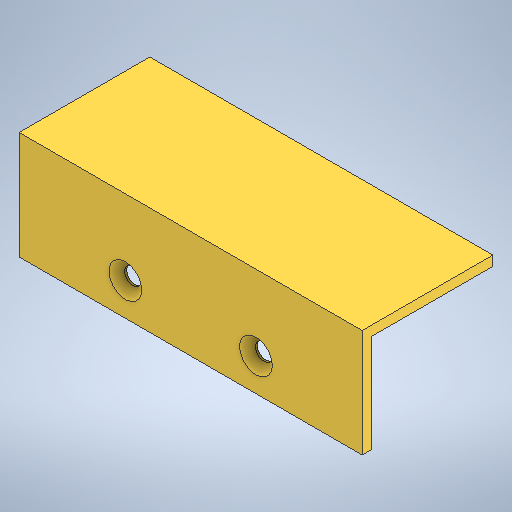
# Autodesk Inventor part: TS_Magazin_Begrenzung_int
Saved by Autodesk Inventor 2025.2 (Build 292293000, 293)
## iProperties
Created: 2025-06-01
Part Number: TS_Magazin_Begrenzung_int
Material: Generisch
Document SubType Name: Modeling
Designer: tino
Density: 1 g/cm^3
Appearance: Vorgabe
Author: tino
Autodesk Inventor part; units mm, degrees
ref_plane "YZ Plane" through (0, 0, 0) normal (1, 0, 0) x (0, 1, 0)
ref_plane "XZ Plane" through (0, 0, 0) normal (0, 1, 0) x (-1, 0, 0)
ref_plane "XY Plane" through (0, 0, 0) normal (0, 0, 1) x (1, 0, 0)
sketch "Skizze1" plane through (0, 0, 0) normal (1, 0, 0) x (0, 1, 0)
  line L0 (0, 0) -> (3, 0)
  line L1 (3, 0) -> (3, 30)
  line L2 (3, 30) -> (0, 30)
  line L3 (0, 30) -> (0, 0)
  line L4 (0, 30) -> (40, 30)
  line L5 (40, 30) -> (40, 33)
  line L6 (40, 33) -> (0, 33)
  line L7 (0, 33) -> (0, 30)
  dimension "d1" = 3
  dimension "d2" = 30
  dimension "d3" = 40
  dimension "d4" = 3
  constraints: 16 end point, 4 parallel, 2 horizontal, 2 perpendicular
  measures "d1" distance of L2.end L1.end
  measures "d2" distance of L1.end L0.end
  measures "d3" distance of L6.end L5.end
  measures "d4" distance between parallel lines of L4 L6
extrude "Extrusion1" add sketch "Skizze1" along normal mid plane 105
sketch "Skizze2" plane through (-52.5, 0, 0) normal (0, -1, 0) x (1, 0, 0)
  line L0 (10.5897, 10) -> (79.1743, 10) construction
  line L1 (0, 0) -> (105, 0) construction
  line L2 (52.5, 0) -> (52.5, 22.0905) construction
  point P0 (32.5, 10)
  point P1 (72.5, 10)
  dimension "d7" = 10
  dimension "d8" = 20
  constraints: 4 end point, 1 horizontal, 1 point on line, 1 symmetric about line, 1 vertical
  measures "d7" distance between parallel lines of L1 L0
  measures "d8" distance from line of point (32.5, 10) L2
hole "Bohrung1" at (-20, 0, 10) at (20, 0, 10) direction (0, 1, 0) diameter 5.2 end through all countersink diameter 10 countersink angle 90
equation "\"d5\" = Magazin_Breite"
equation "\"Magazin_Breite\" = 105"
